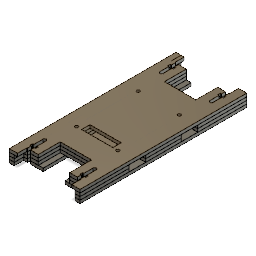
Master Base Mount v6 (Autodesk Fusion 360 design; units mm, degrees)
Autodesk Fusion 360 part; units mm, degrees
note: some values were not read from the file. Set by a fixed rule: which sketch regions a step uses.
sketch "Sketch1" plane through (0, 0, 0) normal (0, 1, 0) x (1, 0, 0)
  line L0 (34, 80) -> (-34, 80)
  line L1 (-34, 80) -> (-34, -80)
  line L2 (-34, -80) -> (34, -80)
  line L3 (34, -80) -> (34, 80)
  line L4 (34, 80) -> (-34, -80) construction
  line L5 (-34, 80) -> (34, -80) construction
  line L6 (-10.2206, 80) -> (-10.3602, 40.0362)
  arc A0 (-10.3602, 40.0362) -> (10.3602, 39.9638) centre (0, 40) ccw
  line L7 (10.3602, 39.9638) -> (10.5, 80)
  line L8 (0, 80) -> (0, 40) construction
  line L9 (-34, 0) -> (34, 0) construction
  line L10 (-10.2206, -80) -> (-10.3602, -40.0362)
  line L11 (10.3602, -39.9638) -> (10.5, -80)
  arc A1 (10.3602, -39.9638) -> (-10.3602, -40.0362) centre (0, -40) ccw
  line L12 (0, -80) -> (0, -40) construction
  line L13 (22.5, 80) -> (22.5, 56)
  arc A2 (22.5, 56) -> (25.5, 56) centre (24, 56) ccw
  line L14 (25.5, 56) -> (25.5, 80)
  arc A3 (25.5, 80) -> (22.5, 80) centre (24, 80) ccw
  line L15 (24, 80) -> (24, 56) construction
  line L16 (26.675, 64.875) -> (21.325, 64.875)
  line L17 (21.325, 64.875) -> (21.325, 67.125)
  line L18 (21.325, 67.125) -> (26.675, 67.125)
  line L19 (26.675, 67.125) -> (26.675, 64.875)
  line L20 (26.675, 64.875) -> (21.325, 67.125) construction
  line L21 (21.325, 64.875) -> (26.675, 67.125) construction
  line L22 (-25.5, 56) -> (-25.5, 80)
  line L23 (-22.5, 80) -> (-22.5, 56)
  line L24 (-21.325, 67.125) -> (-26.675, 67.125)
  line L25 (-21.325, 64.875) -> (-21.325, 67.125)
  line L26 (-26.675, 67.125) -> (-26.675, 64.875)
  arc A4 (-25.5, 56) -> (-22.5, 56) centre (-24, 56) ccw
  line L27 (-26.675, 64.875) -> (-21.325, 64.875)
  line L28 (-22.5, -80) -> (-22.5, -56)
  line L29 (-25.5, -56) -> (-25.5, -80)
  line L30 (-21.325, -67.125) -> (-26.675, -67.125)
  line L31 (-26.675, -64.875) -> (-21.325, -64.875)
  line L32 (-26.675, -67.125) -> (-26.675, -64.875)
  line L33 (-21.325, -64.875) -> (-21.325, -67.125)
  arc A5 (-22.5, -56) -> (-25.5, -56) centre (-24, -56) ccw
  arc A6 (25.5, -56) -> (22.5, -56) centre (24, -56) ccw
  line L34 (25.5, -56) -> (25.5, -80)
  line L35 (22.5, -80) -> (22.5, -56)
  line L36 (26.675, -64.875) -> (21.325, -64.875)
  line L37 (21.325, -67.125) -> (26.675, -67.125)
  line L38 (26.675, -67.125) -> (26.675, -64.875)
  line L39 (21.325, -64.875) -> (21.325, -67.125)
  line L40 (28.9997, 71) -> (-28.9911, 71)
  line L41 (-28.9911, 71) -> (-29, 80)
  line L42 (29, 80) -> (28.9997, 71)
  line L43 (-28.9911, -71) -> (-29, -80)
  line L44 (28.9997, -71) -> (-28.9911, -71)
  line L45 (29, -80) -> (28.9997, -71)
  point P0 (24, 66)
  dimension "d1" = 160
  dimension "d2" = 68
  dimension "d6" = 3
  dimension "d7" = 24
  dimension "d8" = 2.25
  dimension "d9" = 5.35
  dimension "d10" = 14
  dimension "d11" = 24
  dimension "d29" = 40
  dimension "d54" = 9
  dimension "d55" = 9
  dimension "d56" = 10.5
  measures "d1" distance of L0.end L1.end
  measures "d2" distance of L1.end L2.end
  measures "d6" diameter of A2
  measures "d7" distance of L8 L15
  measures "d8" distance of L16.end L17.end
  measures "d9" distance of L16.start L16.end
  measures "d10" distance of L0 P0
  measures "d11" distance of A3.centre A2.centre
  measures "d29" distance of L0 A0.centre
  measures "d54" distance of L40.start L42.start
  measures "d55" distance of L40.end L41.end
  measures "d56" distance of L7.end L8.start
extrude "Extrude1" add sketch "Sketch1" along normal blind 3 contours L0 L1 L2 L3 L6 A0 L7 L10 L11 A1 L13 A2 L14 L16 L17 L18 L19 L22 L23 L24 L25 L26 A4 L27 L28 L29 L30 L31 L32 L33 A5 A6 L34 L35 L36 L37 L38 L39 L40 L41 L42 L43 L44 L45 makes body 1
ref_plane "WorkPlane1" through (0, 3, 0) normal (0, 1, 0) x (1, 0, 0)
sketch "Sketch2" plane through (0, 3, 0) normal (0, 1, 0) x (1, 0, 0)
  line L0 (29, -80) -> (34, -80)
  line L1 (34, -80) -> (34, 80)
  line L2 (34, 80) -> (29, 80)
  line L3 (29, 80) -> (28.9997, 71)
  line L4 (28.9997, 71) -> (25.5, 71)
  line L5 (25.5, 71) -> (25.5, 67.125)
  line L6 (25.5, 67.125) -> (26.675, 67.125)
  line L7 (26.675, 67.125) -> (26.675, 64.875)
  line L8 (26.675, 64.875) -> (25.5, 64.875)
  line L9 (25.5, 64.875) -> (25.5, 56)
  arc A0 (22.5, 56) -> (25.5, 56) centre (24, 56) ccw
  line L10 (22.5, 56) -> (22.5, 64.875)
  line L11 (22.5, 64.875) -> (21.325, 64.875)
  line L12 (21.325, 64.875) -> (21.325, 67.125)
  line L13 (21.325, 67.125) -> (22.5, 67.125)
  line L14 (22.5, 67.125) -> (22.5, 71)
  line L15 (22.5, 71) -> (10.4686, 71)
  line L16 (10.4686, 71) -> (10.3602, 39.9638)
  arc A1 (-10.3602, 40.0362) -> (10.3602, 39.9638) centre (0, 40) ccw
  line L17 (-10.3602, 40.0362) -> (-10.252, 71)
  line L18 (-10.252, 71) -> (-22.5, 71)
  line L19 (-22.5, 71) -> (-22.5, 67.125)
  line L20 (-22.5, 67.125) -> (-21.325, 67.125)
  line L21 (-21.325, 67.125) -> (-21.325, 64.875)
  line L22 (-21.325, 64.875) -> (-22.5, 64.875)
  line L23 (-22.5, 64.875) -> (-22.5, 56)
  arc A2 (-25.5, 56) -> (-22.5, 56) centre (-24, 56) ccw
  line L24 (-25.5, 56) -> (-25.5, 64.875)
  line L25 (-25.5, 64.875) -> (-26.675, 64.875)
  line L26 (-26.675, 64.875) -> (-26.675, 67.125)
  line L27 (-26.675, 67.125) -> (-25.5, 67.125)
  line L28 (-25.5, 67.125) -> (-25.5, 71)
  line L29 (-25.5, 71) -> (-28.9911, 71)
  line L30 (-28.9911, 71) -> (-29, 80)
  line L31 (-29, 80) -> (-34, 80)
  line L32 (-34, 80) -> (-34, -80)
  line L33 (-34, -80) -> (-29, -80)
  line L34 (-25.5, -71) -> (-25.5, -67.125)
  line L35 (-25.5, -67.125) -> (-26.675, -67.125)
  line L36 (-26.675, -67.125) -> (-26.675, -64.875)
  line L37 (-26.675, -64.875) -> (-25.5, -64.875)
  line L38 (-25.5, -64.875) -> (-25.5, -56)
  arc A3 (-22.5, -56) -> (-25.5, -56) centre (-24, -56) ccw
  line L39 (-22.5, -56) -> (-22.5, -64.875)
  line L40 (-22.5, -64.875) -> (-21.325, -64.875)
  line L41 (-21.325, -64.875) -> (-21.325, -67.125)
  line L42 (-21.325, -67.125) -> (-22.5, -67.125)
  line L43 (-22.5, -67.125) -> (-22.5, -71)
  line L44 (-10.252, -71) -> (-10.3602, -40.0362)
  arc A4 (10.3602, -39.9638) -> (-10.3602, -40.0362) centre (0, -40) ccw
  line L45 (10.3602, -39.9638) -> (10.4686, -71)
  line L46 (22.5, -71) -> (22.5, -67.125)
  line L47 (22.5, -67.125) -> (21.325, -67.125)
  line L48 (21.325, -67.125) -> (21.325, -64.875)
  line L49 (21.325, -64.875) -> (22.5, -64.875)
  line L50 (22.5, -64.875) -> (22.5, -56)
  arc A5 (25.5, -56) -> (22.5, -56) centre (24, -56) ccw
  line L51 (25.5, -56) -> (25.5, -64.875)
  line L52 (25.5, -64.875) -> (26.675, -64.875)
  line L53 (26.675, -64.875) -> (26.675, -67.125)
  line L54 (26.675, -67.125) -> (25.5, -67.125)
  line L55 (25.5, -67.125) -> (25.5, -71)
  line L56 (-34, 80) -> (34, 80)
  line L57 (34, 80) -> (34, -80)
  line L58 (34, -80) -> (-34, -80)
  line L59 (-34, -80) -> (-34, 80)
  line L60 (15, 45) -> (-15, 45)
  line L61 (-15, 45) -> (-15, -45)
  line L62 (-15, -45) -> (15, -45)
  line L63 (15, -45) -> (15, 45)
  line L64 (15, 45) -> (-15, -45) construction
  line L65 (-15, 45) -> (15, -45) construction
  line L66 (29, 12.5) -> (-29, 12.5)
  line L67 (-29, 12.5) -> (-29, -12.5)
  line L68 (-29, -12.5) -> (29, -12.5)
  line L69 (29, -12.5) -> (29, 12.5)
  line L70 (29, 12.5) -> (-29, -12.5) construction
  line L71 (-29, 12.5) -> (29, -12.5) construction
  line L72 (-34, 0) -> (34, 0) construction
  line L73 (-14.9948, 80) -> (15.0052, 80)
  line L74 (15.0052, 80) -> (15.0052, 50)
  line L75 (15.0052, 50) -> (-14.9948, 50)
  line L76 (-14.9948, 50) -> (-14.9948, 80)
  line L77 (15.0052, -80) -> (15.0052, -50)
  line L78 (-14.9948, -50) -> (-14.9948, -80)
  line L79 (15.0052, -50) -> (-14.9948, -50)
  line L80 (0, 25) -> (0, -25) construction
  line L81 (-34, 33) -> (-24, 33)
  line L82 (-24, 33) -> (-24, 17)
  line L83 (-24, 17) -> (-34, 17)
  line L84 (-34, 17) -> (-34, 33)
  line L85 (-34, 25) -> (-24, 25) construction
  line L86 (34, 33) -> (24, 33)
  line L87 (24, 33) -> (24, 17)
  line L88 (24, 17) -> (34, 17)
  line L89 (34, 25) -> (24, 25) construction
  line L90 (34, -33) -> (24, -33)
  line L91 (24, -33) -> (24, -17)
  line L92 (24, -17) -> (34, -17)
  line L93 (34, -25) -> (24, -25) construction
  line L94 (-24, -33) -> (-24, -17)
  line L95 (-34, -33) -> (-24, -33)
  line L96 (-34, -25) -> (-24, -25) construction
  line L97 (-24, -17) -> (-34, -17)
  line L98 (-14.9948, -50) -> (-14.9948, -80)
  line L99 (15.0052, -80) -> (15.0052, -50)
  line L100 (15.0052, -50) -> (-14.9948, -50)
  line L101 (-29, -80) -> (-28.9911, -71)
  line L102 (-28.9911, -71) -> (-25.5, -71)
  line L103 (-22.5, -71) -> (-10.252, -71)
  line L104 (10.4686, -71) -> (22.5, -71)
  line L105 (25.5, -71) -> (28.9997, -71)
  line L106 (28.9997, -71) -> (29, -80)
  dimension "d20" = 25
  dimension "d21" = 5
  dimension "d25" = 30
  dimension "d26" = 30
  dimension "d31" = 10
  dimension "d32" = 25
  dimension "d33" = 16
  dimension "d49" = 30
  dimension "d50" = 5
  measures "d20" distance of L66.end L67.end
  measures "d21" distance of L57 L69
  measures "d25" distance of L73.start L73.end
  measures "d26" distance of L73.end L74.end
  measures "d31" distance of L82 L84
  measures "d32" distance of L72 L85
  measures "d33" distance of L81.end L82.end
  measures "d49" distance of L61.end L62.end
  measures "d50" distance of L60 L75
extrude "Extrude2" add sketch "Sketch2" along normal blind 3 separate body contours L0 L1 L2 L3 L4 L5 L6 L7 L8 L9 A0 L10 L11 L12 L13 L14 L15 L16 L45 L46 L47 L48 L49 L50 A5 L51 L52 L53 L54 L55 L56 L57 L58 L60 L62 L63 L66 L68 L69 L74 L75 L77 L79 L86 L87 L88 L90 L91 L92 L99 L100 L104 L105 L106 | L17 L18 L19 L20 L21 L22 L23 A2 L24 L25 L26 L27 L28 L29 L30 L31 L32 L33 L34 L35 L36 L37 L38 A3 L39 L40 L41 L42 L43 L44 L56 L58 L59 L60 L61 L62 L66 L67 L68 L75 L76 L78 L79 L81 L82 L83 L94 L95 L97 L98 L100 L101 L102 L103 | L44 L45 L62 L79 L100 | L16 L17 L60 L75 makes body 2
ref_plane "WorkPlane2" through (0, 6, 0) normal (0, 1, 0) x (1, 0, 0)
sketch "Sketch3" plane through (0, 6, 0) normal (0, 1, 0) x (1, 0, 0)
  line L0 (29, 12.5) -> (29, -12.5)
  line L1 (29, -12.5) -> (15, -12.5)
  line L2 (15, -12.5) -> (15, -45)
  line L3 (15, -45) -> (-15, -45)
  line L4 (-15, -45) -> (-15, -12.5)
  line L5 (-15, -12.5) -> (-29, -12.5)
  line L6 (-29, -12.5) -> (-29, 12.5)
  line L7 (-29, 12.5) -> (-15, 12.5)
  line L8 (-15, 12.5) -> (-15, 45)
  line L9 (-15, 45) -> (15, 45)
  line L10 (15, 45) -> (15, 12.5)
  line L11 (15, 12.5) -> (29, 12.5)
  line L12 (-14.9948, -71) -> (-14.9948, -50)
  line L13 (-14.9948, -50) -> (15.0052, -50)
  line L14 (15.0052, -50) -> (15.0052, -71)
  line L15 (29, -80) -> (34, -80)
  line L16 (34, -80) -> (34, -33)
  line L17 (34, 80) -> (29, 80)
  line L18 (29, 80) -> (28.9997, 71)
  line L19 (28.9997, 71) -> (25.5, 71)
  line L20 (25.5, 71) -> (25.5, 67.125)
  line L21 (25.5, 67.125) -> (26.675, 67.125)
  line L22 (26.675, 67.125) -> (26.675, 64.875)
  line L23 (26.675, 64.875) -> (25.5, 64.875)
  line L24 (25.5, 64.875) -> (25.5, 56)
  arc A0 (22.5, 56) -> (25.5, 56) centre (24, 56) ccw
  line L25 (22.5, 56) -> (22.5, 64.875)
  line L26 (22.5, 64.875) -> (21.325, 64.875)
  line L27 (21.325, 64.875) -> (21.325, 67.125)
  line L28 (21.325, 67.125) -> (22.5, 67.125)
  line L29 (22.5, 67.125) -> (22.5, 71)
  line L30 (22.5, 71) -> (15.0052, 71)
  line L31 (15.0052, 71) -> (15.0052, 50)
  line L32 (15.0052, 50) -> (-14.9948, 50)
  line L33 (-14.9948, 50) -> (-14.9948, 71)
  line L34 (-14.9948, 71) -> (-22.5, 71)
  line L35 (-22.5, 71) -> (-22.5, 67.125)
  line L36 (-22.5, 67.125) -> (-21.325, 67.125)
  line L37 (-21.325, 67.125) -> (-21.325, 64.875)
  line L38 (-21.325, 64.875) -> (-22.5, 64.875)
  line L39 (-22.5, 64.875) -> (-22.5, 56)
  arc A1 (-25.5, 56) -> (-22.5, 56) centre (-24, 56) ccw
  line L40 (-25.5, 56) -> (-25.5, 64.875)
  line L41 (-25.5, 64.875) -> (-26.675, 64.875)
  line L42 (-26.675, 64.875) -> (-26.675, 67.125)
  line L43 (-26.675, 67.125) -> (-25.5, 67.125)
  line L44 (-25.5, 67.125) -> (-25.5, 71)
  line L45 (-25.5, 71) -> (-28.9911, 71)
  line L46 (-28.9911, 71) -> (-29, 80)
  line L47 (-29, 80) -> (-34, 80)
  line L48 (-34, 80) -> (-34, 33)
  line L49 (-34, 33) -> (-24, 33)
  line L50 (-24, 33) -> (-24, 17)
  line L51 (-24, 17) -> (-34, 17)
  line L52 (-34, 17) -> (-34, -17)
  line L53 (-34, -17) -> (-24, -17)
  line L54 (-24, -17) -> (-24, -33)
  line L55 (-24, -33) -> (-34, -33)
  line L56 (-34, -33) -> (-34, -80)
  line L57 (-34, -80) -> (-29, -80)
  line L58 (34, -33) -> (24, -33)
  line L59 (24, -33) -> (24, -17)
  line L60 (24, -17) -> (34, -17)
  line L61 (34, -17) -> (34, 17)
  line L62 (34, 17) -> (24, 17)
  line L63 (24, 17) -> (24, 33)
  line L64 (24, 33) -> (34, 33)
  line L65 (34, 33) -> (34, 80)
  line L66 (25.5, -56) -> (25.5, -64.875)
  line L67 (25.5, -64.875) -> (26.675, -64.875)
  line L68 (26.675, -64.875) -> (26.675, -67.125)
  line L69 (26.675, -67.125) -> (25.5, -67.125)
  line L70 (25.5, -67.125) -> (25.5, -71)
  line L71 (25.5, -71) -> (28.9997, -71)
  line L72 (28.9997, -71) -> (29, -80)
  line L73 (-29, -80) -> (-28.9911, -71)
  line L74 (-28.9911, -71) -> (-25.5, -71)
  line L75 (-25.5, -71) -> (-25.5, -67.125)
  line L76 (-25.5, -67.125) -> (-26.675, -67.125)
  line L77 (-26.675, -67.125) -> (-26.675, -64.875)
  line L78 (-26.675, -64.875) -> (-25.5, -64.875)
  line L79 (-25.5, -64.875) -> (-25.5, -56)
  arc A2 (-22.5, -56) -> (-25.5, -56) centre (-24, -56) ccw
  line L80 (-22.5, -56) -> (-22.5, -64.875)
  line L81 (-22.5, -64.875) -> (-21.325, -64.875)
  line L82 (-21.325, -64.875) -> (-21.325, -67.125)
  line L83 (-21.325, -67.125) -> (-22.5, -67.125)
  line L84 (-22.5, -67.125) -> (-22.5, -71)
  line L85 (-22.5, -71) -> (-14.9948, -71)
  line L86 (15.0052, -71) -> (22.5, -71)
  line L87 (22.5, -71) -> (22.5, -67.125)
  line L88 (22.5, -67.125) -> (21.325, -67.125)
  line L89 (21.325, -67.125) -> (21.325, -64.875)
  line L90 (21.325, -64.875) -> (22.5, -64.875)
  line L91 (22.5, -64.875) -> (22.5, -56)
  arc A3 (25.5, -56) -> (22.5, -56) centre (24, -56) ccw
extrude "Extrude3" add sketch "Sketch3" along normal blind 3 separate body makes body 3
ref_plane "WorkPlane3" through (0, 9, 0) normal (0, 1, 0) x (1, 0, 0)
sketch "Sketch4" plane through (0, 9, 0) normal (0, 1, 0) x (1, 0, 0)
  line L0 (15, 45) -> (15, 12.5)
  line L1 (15, 12.5) -> (29, 12.5)
  line L2 (29, 12.5) -> (29, -12.5)
  line L3 (29, -12.5) -> (15, -12.5)
  line L4 (15, -12.5) -> (15, -45)
  line L5 (15, -45) -> (-15, -45)
  line L6 (-15, -45) -> (-15, -12.5)
  line L7 (-15, -12.5) -> (-29, -12.5)
  line L8 (-29, -12.5) -> (-29, 12.5)
  line L9 (-29, 12.5) -> (-15, 12.5)
  line L10 (-15, 12.5) -> (-15, 45)
  line L11 (-15, 45) -> (15, 45)
  line L12 (-25.5, 56) -> (-25.5, 64.875)
  line L13 (-25.5, 64.875) -> (-26.675, 64.875)
  line L14 (-26.675, 64.875) -> (-26.675, 67.125)
  line L15 (-26.675, 67.125) -> (-25.5, 67.125)
  line L16 (-25.5, 67.125) -> (-25.5, 71)
  line L17 (-25.5, 71) -> (-28.9911, 71)
  line L18 (-28.9911, 71) -> (-29, 80)
  line L19 (-29, 80) -> (-34, 80)
  line L20 (-34, 80) -> (-34, 33)
  line L21 (-34, 33) -> (-24, 33)
  line L22 (-24, 33) -> (-24, 17)
  line L23 (-24, 17) -> (-34, 17)
  line L24 (-34, 17) -> (-34, -17)
  line L25 (-34, -17) -> (-24, -17)
  line L26 (-24, -17) -> (-24, -33)
  line L27 (-24, -33) -> (-34, -33)
  line L28 (-34, -33) -> (-34, -80)
  line L29 (-34, -80) -> (-29, -80)
  line L30 (-14.9948, -71) -> (-14.9948, -50)
  line L31 (-14.9948, -50) -> (15.0052, -50)
  line L32 (15.0052, -50) -> (15.0052, -71)
  line L33 (29, -80) -> (34, -80)
  line L34 (34, -80) -> (34, -33)
  line L35 (34, 80) -> (29, 80)
  line L36 (29, 80) -> (28.9997, 71)
  line L37 (28.9997, 71) -> (25.5, 71)
  line L38 (25.5, 71) -> (25.5, 67.125)
  line L39 (25.5, 67.125) -> (26.675, 67.125)
  line L40 (26.675, 67.125) -> (26.675, 64.875)
  line L41 (26.675, 64.875) -> (25.5, 64.875)
  line L42 (25.5, 64.875) -> (25.5, 56)
  arc A0 (22.5, 56) -> (25.5, 56) centre (24, 56) ccw
  line L43 (22.5, 56) -> (22.5, 64.875)
  line L44 (22.5, 64.875) -> (21.325, 64.875)
  line L45 (21.325, 64.875) -> (21.325, 67.125)
  line L46 (21.325, 67.125) -> (22.5, 67.125)
  line L47 (22.5, 67.125) -> (22.5, 71)
  line L48 (22.5, 71) -> (15.0052, 71)
  line L49 (15.0052, 71) -> (15.0052, 50)
  line L50 (15.0052, 50) -> (-14.9948, 50)
  line L51 (-14.9948, 50) -> (-14.9948, 71)
  line L52 (-14.9948, 71) -> (-22.5, 71)
  line L53 (-22.5, 71) -> (-22.5, 67.125)
  line L54 (-22.5, 67.125) -> (-21.325, 67.125)
  line L55 (-21.325, 67.125) -> (-21.325, 64.875)
  line L56 (-21.325, 64.875) -> (-22.5, 64.875)
  line L57 (-22.5, 64.875) -> (-22.5, 56)
  arc A1 (-25.5, 56) -> (-22.5, 56) centre (-24, 56) ccw
  line L58 (19.75, 29.5) -> (-19.75, 29.5) construction
  line L59 (-19.75, 29.5) -> (-19.75, -29.5) construction
  line L60 (-19.75, -29.5) -> (19.75, -29.5) construction
  line L61 (19.75, -29.5) -> (19.75, 29.5) construction
  line L62 (19.75, 29.5) -> (-19.75, -29.5) construction
  line L63 (-19.75, 29.5) -> (19.75, -29.5) construction
  circle A2 centre (-19.75, 29.5) radius 1.5
  circle A3 centre (19.75, 29.5) radius 1.5
  circle A4 centre (19.75, -29.5) radius 1.5
  circle A5 centre (-19.75, -29.5) radius 1.5
  line L64 (-29, 80) -> (-26, 80)
  line L65 (-26, 80) -> (-26, 71)
  line L66 (-26, 71) -> (-29, 71)
  line L67 (-29, 71) -> (-29, 80)
  line L68 (-34, 0) -> (34, 0) construction
  line L69 (0.0052, 50) -> (0.0052, -50) construction
  line L70 (29.0105, 80) -> (26.0105, 80)
  line L71 (26.0105, 80) -> (26.0105, 71)
  line L72 (-15, -29.5) -> (15, -29.5)
  line L73 (15, -29.5) -> (15, -21.5)
  line L74 (15, -21.5) -> (-15, -21.5)
  line L75 (-15, -21.5) -> (-15, -29.5)
  line L76 (-34, 33) -> (-34, 17)
  line L77 (-34, -17) -> (-34, -33)
  line L78 (34, -33) -> (24, -33)
  line L79 (24, -33) -> (24, -17)
  line L80 (24, -17) -> (34, -17)
  line L81 (34, -17) -> (34, 17)
  line L82 (34, 17) -> (24, 17)
  line L83 (24, 17) -> (24, 33)
  line L84 (24, 33) -> (34, 33)
  line L85 (34, 33) -> (34, 80)
  line L86 (34, 33) -> (34, 17)
  line L87 (34, -17) -> (34, -33)
  line L88 (-29, -80) -> (-26, -80)
  line L89 (-26, -80) -> (-26, -71)
  line L90 (26.0105, -80) -> (26.0105, -71)
  line L91 (29.0105, -80) -> (26.0105, -80)
  line L92 (25.5, -64.875) -> (26.675, -64.875)
  line L93 (26.675, -64.875) -> (26.675, -67.125)
  line L94 (26.675, -67.125) -> (25.5, -67.125)
  line L95 (25.5, -67.125) -> (25.5, -71)
  line L96 (25.5, -71) -> (28.9997, -71)
  line L97 (28.9997, -71) -> (29, -80)
  line L98 (-29, -80) -> (-28.9911, -71)
  line L99 (-28.9911, -71) -> (-25.5, -71)
  line L100 (-25.5, -71) -> (-25.5, -67.125)
  line L101 (-25.5, -67.125) -> (-26.675, -67.125)
  line L102 (-26.675, -67.125) -> (-26.675, -64.875)
  line L103 (-26.675, -64.875) -> (-25.5, -64.875)
  line L104 (-25.5, -64.875) -> (-25.5, -56)
  arc A6 (-22.5, -56) -> (-25.5, -56) centre (-24, -56) ccw
  line L105 (-22.5, -56) -> (-22.5, -64.875)
  line L106 (-22.5, -64.875) -> (-21.325, -64.875)
  line L107 (-21.325, -64.875) -> (-21.325, -67.125)
  line L108 (-21.325, -67.125) -> (-22.5, -67.125)
  line L109 (-22.5, -67.125) -> (-22.5, -71)
  line L110 (-22.5, -71) -> (-14.9948, -71)
  line L111 (15.0052, -71) -> (22.5, -71)
  line L112 (22.5, -71) -> (22.5, -67.125)
  line L113 (22.5, -67.125) -> (21.325, -67.125)
  line L114 (21.325, -67.125) -> (21.325, -64.875)
  line L115 (21.325, -64.875) -> (22.5, -64.875)
  line L116 (22.5, -64.875) -> (22.5, -56)
  arc A7 (25.5, -56) -> (22.5, -56) centre (24, -56) ccw
  line L117 (25.5, -56) -> (25.5, -64.875)
  dimension "d38" = 59
  dimension "d39" = 39.5
  dimension "d40" = 3
  dimension "d41" = 3
  dimension "d42" = 3
  dimension "d43" = 3
  dimension "d46" = 3
  dimension "d47" = 8
  measures "d38" distance of L58.end L59.end
  measures "d39" distance of L59.end L60.end
  measures "d40" diameter of A2
  measures "d41" diameter of A3
  measures "d42" diameter of A4
  measures "d43" diameter of A5
  measures "d46" distance of L65 L67
  measures "d47" distance of L72.start L74.end
extrude "Extrude5" cut sketch "Sketch4" against normal through all contours A2 | A3 | A4 | A5 bodies 1 2 3
extrude "Extrude4" add sketch "Sketch4" along normal blind 3 separate body contours L0 L1 L2 L3 L4 L6 L7 L8 L9 L10 L11 L74 | L4 L5 L6 L72 | L12 L13 L14 L15 L16 L17 L19 L20 L21 L22 L23 L24 L25 L26 L27 L28 L29 L30 L31 L32 L33 L34 L35 L36 L37 L38 L39 L40 L41 L42 A0 L43 L44 L45 L46 L47 L48 L49 L50 L51 L52 L53 L54 L55 L56 L57 A1 L66 L67 L70 L78 L79 L80 L81 L82 L83 L84 L85 L91 L92 L93 L94 L95 L96 L97 L98 L99 L100 L101 L102 L103 L104 A6 L105 L106 L107 L108 L109 L110 L111 L112 L113 L114 L115 L116 A7 L117 | L17 L18 L64 L65 L66 | L21 L22 L23 L76 | L25 L26 L27 L77 | L88 L89 L98 L99 | L36 L37 L70 L71 | L82 L83 L84 L86 | L78 L79 L80 L87 | L90 L91 L96 L97 makes body 4
sketch "Sketch6" plane through (0, 12, 0) normal (0, 1, 0) x (-1, 0, 0)
  circle A0 centre (-19.75, 29.5) radius 1.5
  circle A1 centre (-19.75, -29.5) radius 1.5
  circle A2 centre (19.75, 29.5) radius 1.5
  circle A3 centre (19.75, -29.5) radius 1.5
  line L0 (15, 29.5) -> (15, 21.5)
  line L1 (15, 21.5) -> (-15, 21.5)
  line L2 (-15, 21.5) -> (-15, 29.5)
  line L3 (-15, 29.5) -> (15, 29.5)
  line L4 (28.9911, -71) -> (29, -71)
  line L5 (29, -71) -> (29, -80)
  line L6 (29, -80) -> (34, -80)
  line L7 (34, -80) -> (34, 80)
  line L8 (34, 80) -> (26, 80)
  line L9 (26, 80) -> (26, 71)
  line L10 (26, 71) -> (25.5, 71)
  line L11 (25.5, 71) -> (25.5, 67.125)
  line L12 (25.5, 67.125) -> (26.675, 67.125)
  line L13 (26.675, 67.125) -> (26.675, 64.875)
  line L14 (26.675, 64.875) -> (25.5, 64.875)
  line L15 (25.5, 64.875) -> (25.5, 56)
  arc A4 (22.5, 56) -> (25.5, 56) centre (24, 56) ccw
  line L16 (22.5, 56) -> (22.5, 64.875)
  line L17 (22.5, 64.875) -> (21.325, 64.875)
  line L18 (21.325, 64.875) -> (21.325, 67.125)
  line L19 (21.325, 67.125) -> (22.5, 67.125)
  line L20 (22.5, 67.125) -> (22.5, 71)
  line L21 (22.5, 71) -> (14.9948, 71)
  line L22 (14.9948, 71) -> (14.9948, 50)
  line L23 (14.9948, 50) -> (-15.0052, 50)
  line L24 (-15.0052, 50) -> (-15.0052, 71)
  line L25 (-15.0052, 71) -> (-22.5, 71)
  line L26 (-22.5, 71) -> (-22.5, 67.125)
  line L27 (-22.5, 67.125) -> (-21.325, 67.125)
  line L28 (-21.325, 67.125) -> (-21.325, 64.875)
  line L29 (-21.325, 64.875) -> (-22.5, 64.875)
  line L30 (-22.5, 64.875) -> (-22.5, 56)
  arc A5 (-25.5, 56) -> (-22.5, 56) centre (-24, 56) ccw
  line L31 (-25.5, 56) -> (-25.5, 64.875)
  line L32 (-25.5, 64.875) -> (-26.675, 64.875)
  line L33 (-26.675, 64.875) -> (-26.675, 67.125)
  line L34 (-26.675, 67.125) -> (-25.5, 67.125)
  line L35 (-25.5, 67.125) -> (-25.5, 71)
  line L36 (-25.5, 71) -> (-26.0105, 71)
  line L37 (-26.0105, 71) -> (-26.0105, 80)
  line L38 (-26.0105, 80) -> (-34, 80)
  line L39 (-34, 80) -> (-34, -80)
  line L40 (-34, -80) -> (-26.0105, -80)
  line L41 (-26.0105, -80) -> (-26.0105, -71)
  line L42 (-26.0105, -71) -> (-25.5, -71)
  line L43 (-25.5, -71) -> (-25.5, -67.125)
  line L44 (-25.5, -67.125) -> (-26.675, -67.125)
  line L45 (-26.675, -67.125) -> (-26.675, -64.875)
  line L46 (-26.675, -64.875) -> (-25.5, -64.875)
  line L47 (-25.5, -64.875) -> (-25.5, -56)
  arc A6 (-22.5, -56) -> (-25.5, -56) centre (-24, -56) ccw
  line L48 (-22.5, -56) -> (-22.5, -64.875)
  line L49 (-22.5, -64.875) -> (-21.325, -64.875)
  line L50 (-21.325, -64.875) -> (-21.325, -67.125)
  line L51 (-21.325, -67.125) -> (-22.5, -67.125)
  line L52 (-22.5, -67.125) -> (-22.5, -71)
  line L53 (-22.5, -71) -> (-15.0052, -71)
  line L54 (-15.0052, -71) -> (-15.0052, -50)
  line L55 (-15.0052, -50) -> (14.9948, -50)
  line L56 (14.9948, -50) -> (14.9948, -71)
  line L57 (14.9948, -71) -> (22.5, -71)
  line L58 (22.5, -71) -> (22.5, -67.125)
  line L59 (22.5, -67.125) -> (21.325, -67.125)
  line L60 (21.325, -67.125) -> (21.325, -64.875)
  line L61 (21.325, -64.875) -> (22.5, -64.875)
  line L62 (22.5, -64.875) -> (22.5, -56)
  arc A7 (25.5, -56) -> (22.5, -56) centre (24, -56) ccw
  line L63 (25.5, -56) -> (25.5, -64.875)
  line L64 (25.5, -64.875) -> (26.675, -64.875)
  line L65 (26.675, -64.875) -> (26.675, -67.125)
  line L66 (26.675, -67.125) -> (25.5, -67.125)
  line L67 (25.5, -67.125) -> (25.5, -71)
  line L68 (25.5, -71) -> (26, -71)
  line L69 (26, -71) -> (26, -80)
  line L70 (26, -80) -> (29, -80)
  line L71 (29, -80) -> (28.9911, -71)
move_body "Move1" [suppressed]
move_body "Move2" [suppressed]
move_body "Move3" [suppressed]
equation "d1 = height"
equation "d2 = width"
equation "height = 160 mm"
equation "width = 68 mm"
equation "offset = 0 mm"
equation "d17 = offset"
equation "d34 = offset"
equation "d37 = offset"
